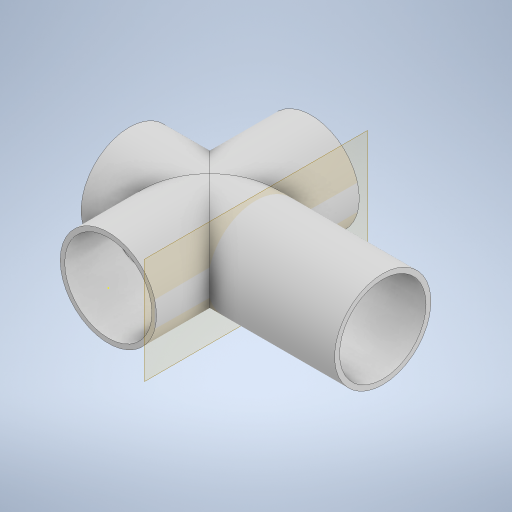
# Autodesk Inventor part: Pieza2
Saved by Autodesk Inventor 2024 (Build 280153000, 153)
## iProperties
Created: 2024-11-05
Part Number: Pieza2
Material: Genérico
Document SubType Name: Modeling
Designer: Aulasedfl
Density: 1 g/cm^3
Appearance: Valor por defecto
Author: Aulasedfl
Autodesk Inventor part; units mm, degrees
ref_plane "XZ Plane" through (0, 0, 0) normal (0, 1, 0) x (-1, 0, 0)
ref_plane "XY Plane" through (0, 0, 0) normal (0, 0, 1) x (1, 0, 0)
sketch "Boceto1" plane through (0, 0, 0) normal (0, 0, 1) x (1, 0, 0)
  circle A0 centre (0, 0) radius 95
  dimension "d0" = 190
  constraints: 1 centre point, 1 coincident
  measures "d0" diameter of A0
extrude "Extrusión1" add sketch "Boceto1" along normal blind 400
sketch "Boceto2" plane through (0, 0, 400) normal (0, 0, 1) x (1, 0, 0)
  point P0 (0, 0)
sketch "Boceto3" plane through (0, 0, 400) normal (0, 0, 1) x (1, 0, 0)
  circle A0 centre (0, 0) radius 86.0432
  constraints: 1 centre point, 1 coincident
extrude "Extrusión2" cut sketch "Boceto3" against normal blind 400
ref_plane "Plano de trabajo2" through (91.25, 0, 0) normal (1, 0, 0) x (0, 1, 0)
sketch "Boceto4" plane through (91.25, 0, 0) normal (1, 0, 0) x (0, 1, 0)
  line L0 (95, 400) -> (-95, 400) construction
  line L1 (0, 400) -> (0, 0) construction
  line L2 (0, 0) -> (0, 400) construction
  line L3 (0, 400) -> (0, 200) construction
  line L4 (95, 0) -> (95, 400) construction
  line L5 (95, 203.9147) -> (-95, 203.9147) construction
  line L6 (-95, 0) -> (-95, 400) construction
  circle A0 centre (0, 200) radius 95
  dimension "d7" = 190
  constraints: 8 end point, 2 midpoint, 2 point on line, 2 vertical, 1 centre point, 1 coincident, 1 perpendicular
  measures "d7" diameter of A0
extrude "Extrusión3" add sketch "Boceto4" along normal mid plane 500
sketch "Boceto5" plane through (0, 0, 400) normal (0, 0, 1) x (1, 0, 0)
  circle A0 centre (0, 0) radius 85.3099
  constraints: 1 centre point, 1 coincident
extrude "Extrusión4" cut sketch "Boceto5" against normal blind 500
sketch "Boceto6" plane through (341.25, 0, 200) normal (1, 0, 0) x (0, 0, -1)
  circle A0 centre (0, 0) radius 85.3099
  line L0 (-41.7999, 85.3099) -> (41.7999, 85.3099) projected
  point P0 (200, 0)
  constraints: 1 centre point, 1 tangent
extrude "Extrusión5" cut sketch "Boceto6" against normal blind 500
